Autodesk Fusion 360 part; units mm, degrees
(part 2 of 3)
  line L576 (512.1919, -690.0793) -> (454.1919, -690.0793)
  line L577 (454.1919, -748.0793) -> (512.1919, -690.0793) construction
  line L578 (527.085, -748.0793) -> (585.085, -748.0793)
  line L579 (512.1919, -748.0793) -> (454.1919, -690.0793) construction
  line L580 (513.1919, -749.0793) -> (526.085, -749.0793) construction
  line L581 (454.1919, -748.0793) -> (512.1919, -748.0793)
  line L582 (585.085, -748.0793) -> (585.085, -690.0793)
  line L583 (381.2987, -690.0793) -> (381.2987, -748.0793)
  line L584 (381.2987, -748.0793) -> (439.2987, -748.0793)
  line L585 (454.1919, -690.0793) -> (454.1919, -748.0793)
  line L586 (527.085, -748.0793) -> (585.085, -690.0793) construction
  line L587 (585.085, -690.0793) -> (527.085, -690.0793)
  line L588 (439.2987, -690.0793) -> (381.2987, -690.0793)
  line L589 (381.2987, -748.0793) -> (439.2987, -690.0793) construction
  line L590 (440.2987, -749.0793) -> (453.1919, -749.0793) construction
  line L591 (585.085, -748.0793) -> (527.085, -690.0793) construction
  line L592 (527.085, -690.0793) -> (527.085, -748.0793)
  line L593 (512.1919, -748.0793) -> (512.1919, -690.0793)
  line L594 (439.2987, -748.0793) -> (381.2987, -690.0793) construction
  line L595 (439.2987, -748.0793) -> (439.2987, -690.0793)
  line L596 (225.4513, -1098.8293) -> (283.4513, -1040.8293) construction
  line L597 (152.5581, -1098.8293) -> (152.5581, -1040.8293)
  line L598 (79.665, -1098.8293) -> (79.665, -1040.8293)
  line L599 (79.665, -1040.8293) -> (137.665, -1040.8293)
  line L600 (137.665, -1098.8293) -> (79.665, -1040.8293) construction
  line L601 (152.5581, -1040.8293) -> (210.5581, -1040.8293)
  line L602 (151.5581, -1099.8293) -> (138.665, -1099.8293) construction
  line L603 (137.665, -1040.8293) -> (137.665, -1098.8293)
  line L604 (79.665, -1098.8293) -> (137.665, -1040.8293) construction
  line L605 (152.5581, -1098.8293) -> (210.5581, -1040.8293) construction
  line L606 (210.5581, -1098.8293) -> (152.5581, -1098.8293)
  line L607 (210.5581, -1098.8293) -> (152.5581, -1040.8293) construction
  line L608 (137.665, -1098.8293) -> (79.665, -1098.8293)
  line L609 (210.5581, -1040.8293) -> (210.5581, -1098.8293)
  line L610 (225.4513, -1098.8293) -> (225.4513, -1040.8293)
  line L611 (283.4513, -1098.8293) -> (225.4513, -1098.8293)
  line L612 (225.4513, -1040.8293) -> (283.4513, -1040.8293)
  line L613 (283.4513, -1040.8293) -> (283.4513, -1098.8293)
  line L614 (283.4513, -1098.8293) -> (225.4513, -1040.8293) construction
  line L615 (224.4513, -1099.8293) -> (211.5581, -1099.8293) construction
  line L616 (332, -925) -> (332, -1216) construction
  line L617 (526.335, -1098.8293) -> (584.335, -1098.8293)
  line L618 (526.335, -1040.8293) -> (526.335, -1098.8293)
  line L619 (526.335, -1098.8293) -> (584.335, -1040.8293) construction
  line L620 (380.5487, -1040.8293) -> (380.5487, -1098.8293)
  line L621 (380.5487, -1098.8293) -> (438.5487, -1098.8293)
  line L622 (439.5487, -1099.8293) -> (452.4419, -1099.8293) construction
  line L623 (453.4419, -1040.8293) -> (453.4419, -1098.8293)
  line L624 (438.5487, -1098.8293) -> (380.5487, -1040.8293) construction
  line L625 (438.5487, -1098.8293) -> (438.5487, -1040.8293)
  line L626 (380.5487, -1098.8293) -> (438.5487, -1040.8293) construction
  line L627 (438.5487, -1040.8293) -> (380.5487, -1040.8293)
  line L628 (511.4419, -1098.8293) -> (511.4419, -1040.8293)
  line L629 (584.335, -1098.8293) -> (526.335, -1040.8293) construction
  line L630 (453.4419, -1098.8293) -> (511.4419, -1098.8293)
  line L631 (584.335, -1098.8293) -> (584.335, -1040.8293)
  line L632 (511.4419, -1098.8293) -> (453.4419, -1040.8293) construction
  line L633 (511.4419, -1040.8293) -> (453.4419, -1040.8293)
  line L634 (512.4419, -1099.8293) -> (525.335, -1099.8293) construction
  line L635 (584.335, -1040.8293) -> (526.335, -1040.8293)
  line L636 (453.4419, -1098.8293) -> (511.4419, -1040.8293) construction
  point P0 (-381.2407, -502.1425)
  point P1 (-1045.2407, -502.1425)
  point P2 (332, 4.5)
  point P3 (332, 4.5)
  point P4 (332, -345.5)
  point P5 (332, -345.5)
  point P6 (0, -350)
  point P7 (1200, -500)
  point P8 (1294, -456)
  point P9 (1200, -500)
  point P10 (1200, -412)
  point P11 (1388, -412)
  point P12 (1294, -456)
  point P13 (1755.9968, -408.7804)
  point P14 (1661.9968, -630.2804)
  point P15 (1661.9968, -630.2804)
  point P16 (1567.9968, -496.7804)
  point P17 (1661.9968, -452.7804)
  point P18 (1567.9968, -408.7804)
  point P19 (1661.9968, -452.7804)
  point P20 (1567.9968, -496.7804)
  point P21 (1661.9968, -452.7804)
  point P22 (1781.5009, -1445.9592)
  point P23 (2131.5009, -1445.9592)
  point P24 (2131.5009, -1095.9592)
  point P25 (1781.5009, -1095.9592)
  point P26 (861.9968, -1564.433)
  point P27 (861.9968, -1564.433)
  point P28 (166, -1297.5)
  point P29 (498, -1297.5)
  point P30 (166, -1297.5)
  point P31 (498, -1297.5)
  point P32 (501.8298, -1590.7079)
  point P33 (187.1704, -1945.0478)
  point P34 (501.8298, -1576.2079)
  point P35 (861.9968, -1548.433)
  point P36 (861.9968, -1562.933)
  point P37 (1211.9968, -1564.433)
  point P38 (1211.9968, -1548.433)
  point P39 (1211.9968, -1562.933)
  point P40 (1211.9968, -1564.433)
  point P41 (141.8298, -1576.2079)
  point P42 (141.8298, -1590.7079)
  point P43 (540.3102, -621.1975)
  point P44 (253.7013, -719.0793)
  point P45 (107.915, -719.0793)
  point P46 (123.6898, -621.1975)
  point P47 (107.915, -719.0793)
  point P48 (253.7013, -719.0793)
  point P49 (123.6898, -621.1975)
  point P50 (540.3102, -621.1975)
  point P51 (123.6898, -621.1975)
  point P52 (540.3102, -621.1975)
  point P53 (123.6898, -971.1975)
  point P54 (540.3102, -971.1975)
  point P55 (123.6898, -971.1975)
  point P56 (540.3102, -971.1975)
  point P57 (540.3102, -971.1975)
  point P58 (123.6898, -971.1975)
  point P59 (166, -1297.5)
  point P60 (312.5, -1297.5)
  point P61 (312.5, -1297.5)
  point P62 (107.915, -719.0793)
  point P63 (180.8081, -719.0793)
  point P64 (253.7013, -719.0793)
  point P65 (556.085, -719.0793)
  point P66 (410.2987, -719.0793)
  point P67 (556.085, -719.0793)
  point P68 (410.2987, -719.0793)
  point P69 (410.2987, -719.0793)
  point P70 (483.1919, -719.0793)
  point P71 (556.085, -719.0793)
  point P72 (79.665, -1040.8293)
  point P73 (181.5581, -1069.8293)
  point P74 (108.665, -1069.8293)
  point P75 (254.4513, -1069.8293)
  point P76 (254.4513, -1069.8293)
  point P77 (108.665, -1069.8293)
  point P78 (108.665, -1069.8293)
  point P79 (254.4513, -1069.8293)
  point P80 (482.4419, -1069.8293)
  point P81 (555.335, -1069.8293)
  point P82 (555.335, -1069.8293)
  point P83 (409.5487, -1069.8293)
  point P84 (584.335, -1040.8293)
  point P85 (555.335, -1069.8293)
  point P86 (409.5487, -1069.8293)
  point P87 (409.5487, -1069.8293)
  dimension "d11" = 7
  dimension "d12" = 16.1835
  dimension "d13" = 16.1835
  dimension "d14" = 16.1835
  dimension "d15" = 16.1835
  dimension "d16" = 11.9217
  dimension "d17" = 11.9217
  dimension "d19" = 11.9217
  dimension "d22" = 5.3
  dimension "d23" = 5.3
  dimension "d24" = 5.3
  dimension "d25" = 5.3
  dimension "d26" = 5.3
  dimension "d27" = 22
  dimension "d28" = 22
  dimension "d29" = 22
  dimension "d33" = 5.3
  dimension "d34" = 5.3
  dimension "d35" = 5.3
  dimension "d36" = 5.3
  dimension "d37" = 5.3
  dimension "d38" = 5.3
  dimension "d39" = 5.3
  dimension "d43" = 291
  dimension "d63" = 74.7336
  dimension "d64" = 86
  dimension "d65" = 43
  dimension "d83" = 12.8931
  dimension "d84" = 12.8931
  dimension "d85" = 60
  dimension "d89" = 7
  dimension "d90" = 16.1835
  dimension "d91" = 16.1835
  dimension "d92" = 16.1835
  dimension "d93" = 16.1835
  dimension "d94" = 11.9217
  dimension "d95" = 11.9217
  dimension "d96" = 11.9217
  dimension "d97" = 5.3
  dimension "d98" = 5.3
  dimension "d99" = 5.3
  dimension "d100" = 5.3
  dimension "d101" = 5.3
  dimension "d102" = 22
  dimension "d103" = 22
  dimension "d104" = 22
  dimension "d105" = 5.3
  dimension "d106" = 5.3
  dimension "d107" = 5.3
  dimension "d108" = 5.3
  dimension "d109" = 5.3
  dimension "d110" = 5.3
  dimension "d111" = 5.3
  dimension "d112" = 86
  dimension "d113" = 43
  dimension "d114" = 7
  dimension "d115" = 16.1835
  dimension "d116" = 16.1835
  dimension "d117" = 16.1835
  dimension "d118" = 16.1835
  dimension "d119" = 11.9217
  dimension "d120" = 11.9217
  dimension "d121" = 11.9217
  dimension "d122" = 5.3
  dimension "d123" = 5.3
  dimension "d124" = 5.3
  dimension "d125" = 5.3
  dimension "d126" = 5.3
  dimension "d127" = 22
  dimension "d128" = 22
  dimension "d129" = 22
  dimension "d130" = 5.3
  dimension "d131" = 5.3
  dimension "d132" = 5.3
  dimension "d133" = 5.3
  dimension "d134" = 5.3
  dimension "d135" = 5.3
  dimension "d136" = 5.3
  dimension "d137" = 86
  dimension "d138" = 43
  dimension "d194" = 73
  dimension "d195" = 664
  dimension "d196" = 73
  dimension "d203" = 7
  dimension "d204" = 5.3
  dimension "d205" = 5.3
  dimension "d206" = 5.3
  dimension "d207" = 5.3
  dimension "d208" = 5.3
  dimension "d209" = 5.3
  dimension "d210" = 5.3
  dimension "d211" = 5.3
  dimension "d212" = 5.3
  dimension "d213" = 5.3
  dimension "d214" = 5.3
  dimension "d215" = 5.3
  dimension "d216" = 291
  dimension "d217" = 33
  dimension "d218" = 332
  dimension "d219" = 60
  dimension "d220" = 664
  dimension "d350" = 291
  dimension "d352" = 231
  dimension "d357" = 28.284
  dimension "d358" = 28.284
  dimension "d359" = 28.284
  dimension "d360" = 28.284
  dimension "d361" = 664
  dimension "d362" = 291
  dimension "d363" = 231
  dimension "d364" = 28.284
  dimension "d365" = 28.284
  dimension "d366" = 28.284
  dimension "d367" = 28.284
  dimension "d368" = 30
  dimension "d369" = 30
  dimension "d370" = 30
  dimension "d371" = 30
  dimension "d372" = 30
  dimension "d373" = 30
  dimension "d374" = 30
  dimension "d375" = 30
  dimension "d376" = 6.5
  dimension "d377" = 6.5
  dimension "d378" = 18
  dimension "d379" = 18
  dimension "d380" = 18
  dimension "d381" = 18
  dimension "d382" = 6.5
  dimension "d383" = 6.5
  dimension "d384" = 20
  dimension "d385" = 20
  dimension "d387" = 20
  dimension "d389" = 20
  dimension "d390" = 20
  dimension "d391" = 20
  dimension "d392" = 5
  dimension "d393" = 5
  dimension "d394" = 5
  dimension "d395" = 5
  dimension "d537" = 664
  dimension "d553" = 67
  dimension "d554" = 67
  dimension "d555" = 67
  dimension "d556" = 67
  dimension "d1" = 188
  dimension "d2" = 88
  dimension "d3" = 18
  dimension "d4" = 18
  dimension "d5" = 18
  dimension "d6" = 18
  dimension "d7" = 15
  dimension "d8" = 15
  dimension "d9" = 15
  dimension "d10" = 15
  dimension "d597" = 8
  dimension "d598" = 8
  dimension "d599" = 8
  dimension "d600" = 8
  dimension "d601" = 8
  dimension "d602" = 8
  dimension "d603" = 8
  dimension "d604" = 8
  dimension "d605" = 73
  dimension "d606" = 80
  dimension "d607" = 188
  dimension "d608" = 88
  dimension "d609" = 18
  dimension "d610" = 18
  dimension "d611" = 18
  dimension "d612" = 18
  dimension "d613" = 15
  dimension "d614" = 15
  dimension "d615" = 15
  dimension "d616" = 15
  dimension "d617" = 25
  dimension "d618" = 25
  dimension "d807" = 300
  dimension "d858" = 30
  dimension "d859" = 30
  dimension "d860" = 30
  dimension "d861" = 30
  dimension "d862" = 6.5
  dimension "d863" = 6.5
  dimension "d865" = 6.5
  dimension "d876" = 30
  dimension "d877" = 30
  dimension "d878" = 30
  dimension "d879" = 30
  dimension "d880" = 20
  dimension "d881" = 20
  dimension "d882" = 20
  dimension "d883" = 20
  dimension "d884" = 6.5
  dimension "d892" = 30
  dimension "d893" = 30
  dimension "d894" = 30
  dimension "d895" = 30
  dimension "d896" = 6.5
  dimension "d897" = 6.5
  dimension "d898" = 6.5
  dimension "d899" = 30
  dimension "d900" = 30
  dimension "d901" = 30
  dimension "d902" = 30
  dimension "d903" = 20
  dimension "d904" = 20
  dimension "d905" = 20
  dimension "d906" = 20
  dimension "d907" = 6.5
  dimension "d934" = 300
  dimension "d943" = 25
  dimension "d944" = 25
  dimension "d945" = 20
  dimension "d946" = 20
  dimension "d947" = 20
  dimension "d948" = 20
  dimension "d949" = 20
  dimension "d950" = 20
  dimension "d951" = 20
  dimension "d953" = 5
  dimension "d954" = 5
  dimension "d955" = 5
  dimension "d956" = 5
  dimension "d957" = 300
  dimension "d959" = 20
  dimension "d961" = 20
  dimension "d962" = 20
  dimension "d963" = 20
  dimension "d964" = 20
  dimension "d965" = 20
  dimension "d966" = 5
  dimension "d967" = 5
  dimension "d968" = 5
  dimension "d969" = 5
  dimension "d981" = 37.5
  dimension "d983" = 37.5
  dimension "d1011" = 8
  dimension "d1012" = 8
  dimension "d1013" = 8
  dimension "d1014" = 8
  dimension "d1015" = 8
  dimension "d1016" = 8
  dimension "d1017" = 8
  dimension "d1018" = 29
  dimension "d1019" = 45.5
  dimension "d1020" = 22
  dimension "d1037" = 8
  dimension "d1038" = 8
  dimension "d1039" = 8
  dimension "d1040" = 8
  dimension "d1041" = 8
  dimension "d1042" = 8
  dimension "d1043" = 8
  dimension "d1044" = 29
  dimension "d1045" = 45.5
  dimension "d1046" = 22
  dimension "d1047" = 45.5
  dimension "d1048" = 26.5
  dimension "d1049" = 182
  dimension "d1050" = 29
  dimension "d1051" = 45.5
  dimension "d1052" = 22
  dimension "d1055" = 2.5
  dimension "d1056" = 1.9
  dimension "d1057" = 273
  dimension "d1058" = 73
  dimension "d1059" = 8
  dimension "d1060" = 8
  dimension "d1061" = 8
  dimension "d1062" = 8
  dimension "d1063" = 8
  dimension "d1064" = 8
  dimension "d1065" = 8
  dimension "d1066" = 29
  dimension "d1069" = 182
  dimension "d1072" = 2.5
  dimension "d1073" = 1.9
  dimension "d1074" = 54.5
  dimension "d1075" = 26.5
  dimension "d1076" = 54.5
  dimension "d1077" = 17.5
  dimension "d1094" = 25
  dimension "d1095" = 25
  dimension "d1096" = 8
  dimension "d1097" = 8
  dimension "d1098" = 8
  dimension "d1099" = 8
  dimension "d1100" = 8
  dimension "d1101" = 8
  dimension "d1102" = 8
  dimension "d1103" = 29
  dimension "d1104" = 182
  dimension "d1105" = 2.5
  dimension "d1106" = 1.9
  dimension "d1107" = 54.5
  dimension "d1108" = 26.5
  dimension "d1109" = 54.5
  dimension "d1110" = 26.5
  dimension "d1111" = 8
  dimension "d1112" = 8
  dimension "d1113" = 8
  dimension "d1114" = 8
  dimension "d1115" = 8
  dimension "d1116" = 8
  dimension "d1117" = 8
  dimension "d1118" = 29
  dimension "d1119" = 45.5
  dimension "d1120" = 22
  dimension "d1121" = 182
  dimension "d1122" = 45.5
  dimension "d1123" = 22
  dimension "d1124" = 2.5
  dimension "d1125" = 1.9
  dimension "d1126" = 273
  dimension "d1127" = 73
  dimension "d1144" = 29
  dimension "d1145" = 29
  dimension "d1146" = 29
  dimension "d1147" = 29
  dimension "d1148" = 7
  dimension "d1171" = 291
  dimension "d1174" = 74.7336
  dimension "d1187" = 20
  dimension "d1188" = 20
  dimension "d1189" = 20
  dimension "d1190" = 20
  dimension "d1191" = 20
  dimension "d1192" = 20
  dimension "d1193" = 5
  dimension "d1194" = 5
  dimension "d1195" = 5
  dimension "d1196" = 5
  dimension "d1197" = 664
  dimension "d1210" = 29
  dimension "d1211" = 29
  dimension "d1212" = 29
  dimension "d1213" = 29
  dimension "d1237" = 291
  dimension "d1253" = 20
  dimension "d1254" = 20
  dimension "d1255" = 20
  dimension "d1256" = 20
  dimension "d1257" = 20
  dimension "d1258" = 20
  dimension "d1259" = 5
  dimension "d1260" = 5
  dimension "d1261" = 5
  dimension "d1262" = 5
  dimension "d1263" = 664
  dimension "d1322" = 29
  dimension "d1323" = 29
  dimension "d1324" = 12.5
  dimension "d1325" = 12.5
  dimension "d1326" = 58
  dimension "d1327" = 58
  dimension "d1328" = 58
  dimension "d1329" = 58
  dimension "d1330" = 58
  dimension "d1331" = 58
  dimension "d1332" = 12.8931
  dimension "d1333" = 12.8931
  dimension "d1334" = 60
  dimension "d1335" = 58
  dimension "d1336" = 58
  dimension "d1337" = 58
  dimension "d1338" = 58
  dimension "d1339" = 58
  dimension "d1340" = 58
  constraint horizontal L0
  constraint horizontal L1
  constraint tangent L0 A0
  constraint tangent L1 A0
  constraint tangent L0 A1
  constraint tangent L1 A1
  constraint coincident L0.end A1.end
  constraint vertical L5
  constraint parallel L5 L6
  constraint parallel L6 L7
  constraint vertical L14
  constraint parallel L9 L14
  constraint parallel L9 L13
  constraint tangent A1 L15
  constraint horizontal L16
  constraint vertical L17
  constraint horizontal L19
  constraint vertical L20
  constraint coincident L17.end L18.start
  constraint coincident L20.end L21.end
  constraint coincident L4.end L5.start
  constraint coincident L7.end L8.end
  constraint coincident L22.start A7.centre
  constraint horizontal L23
  constraint parallel L23 L24
  constraint parallel L24 L25
  constraint horizontal L27
  constraint parallel L27 L28
  constraint parallel L28 L29
  constraint coincident L23.end L24.start
  constraint coincident L24.end L25.start
  constraint coincident L25.end A10.centre
  constraint coincident L26.start L27.start
  constraint coincident L27.end L28.start
  constraint coincident L28.end L29.start
  constraint coincident L29.end A14.centre
  constraint horizontal L30
  constraint vertical L31
  constraint horizontal L32
  constraint vertical L33
  constraint horizontal L34
  constraint vertical L35
  constraint vertical L36
  constraint perpendicular L35 L37
  constraint coincident A0.centre L37.end
  constraint horizontal L51
  constraint horizontal L53
  constraint tangent L51 A29
  constraint tangent L53 A29
  constraint tangent A22 L51
  constraint tangent A22 L53
  constraint coincident L42.start A20.end
  constraint vertical L67
  constraint parallel L40 L67
  constraint parallel L40 L44
  constraint vertical L65
  constraint parallel L65 L68
  constraint parallel L66 L68
  constraint tangent L47 A22
  constraint horizontal L56
  constraint vertical L54
  constraint horizontal L60
  constraint vertical L61
  constraint coincident L54.end L58.start
  constraint coincident A27.centre L61.end
  constraint coincident A19.centre L64.end
  constraint coincident L41.end L43.end
  constraint coincident L57.start A26.centre
  constraint horizontal L57
  constraint parallel L52 L57
  constraint parallel L45 L52
  constraint horizontal L46
  constraint parallel L46 L50
  constraint parallel L50 L59
  constraint coincident L52.start L57.end
  constraint coincident A16.centre L45.start
  constraint coincident L45.end A21.centre
  constraint coincident L41.start A17.centre
  constraint coincident A15.centre L46.end
  constraint coincident L50.end A24.centre
  constraint coincident A23.centre L59.end
  constraint coincident L55.end A29.centre
  constraint horizontal L81
  constraint horizontal L79
  constraint tangent A32 L81
  constraint tangent A32 L79
  constraint tangent L81 A37
  constraint tangent L79 A37
  constraint coincident L81.end A37.end
  constraint vertical L71
  constraint parallel L71 L80
  constraint parallel L80 L92
  constraint vertical L88
  constraint parallel L88 L100
  constraint parallel L91 L100
  constraint tangent A37 L84
  constraint horizontal L78
  constraint vertical L93
  constraint horizontal L74
  constraint vertical L75
  constraint coincident A33.centre L93.end
  constraint coincident L72.end L75.end
  constraint coincident L71.start L82.end
  constraint coincident A30.centre L86.end
  constraint coincident L76.start A43.centre
  constraint horizontal L76
  constraint parallel L73 L76
  constraint parallel L73 L85
  constraint horizontal L90
  constraint parallel L90 L95
  constraint parallel L95 L97
  constraint coincident L73.start L76.end
  constraint coincident L73.end L85.start
  constraint coincident A31.centre L85.end
  constraint coincident A36.centre L87.start
  constraint coincident A40.centre L90.end
  constraint coincident L95.end L97.start
  constraint coincident A34.centre L97.end
  constraint coincident A32.centre L96.end
  constraint horizontal L102
  constraint vertical L103
  constraint horizontal L104
  constraint vertical L105
  constraint horizontal L108
  constraint vertical L107
  constraint horizontal L109
  constraint vertical L106
  constraint horizontal L128
  constraint horizontal L127
  constraint tangent A50 L128
  constraint tangent A50 L127
  constraint tangent L128 A59
  constraint tangent L127 A59
  constraint horizontal L136
  constraint vertical L152
  constraint horizontal L139
  constraint vertical L140
  constraint vertical L121
  constraint vertical L129
  constraint horizontal L135
  constraint vertical L130
  constraint horizontal L131
  constraint vertical L138
  constraint horizontal L149
  constraint vertical L142
  constraint horizontal L150
  constraint vertical L147
  constraint horizontal L137
  constraint vertical L134
  constraint horizontal L145
  constraint vertical L143
  constraint horizontal L146
  constraint vertical L151
  constraint perpendicular L143 L144
  constraint horizontal L119
  constraint vertical L126
  constraint horizontal L114
  constraint vertical L148
  constraint perpendicular L111 L126
  constraint horizontal L110
  constraint vertical L154
  constraint horizontal L153
  constraint vertical L155
  constraint horizontal L115
  constraint vertical L117
  constraint horizontal L113
  constraint vertical L124
  constraint horizontal L132
  constraint vertical L112
  constraint horizontal L141
  constraint vertical L123
  constraint horizontal L120
  constraint vertical L125
  constraint horizontal L116
  constraint vertical L122
  constraint horizontal L164
  constraint vertical L156
  constraint horizontal L158
  constraint vertical L157
  constraint horizontal L159
  constraint perpendicular L159 L161
  constraint parallel L159 L163
  constraint parallel L160 L161
  constraint coincident P3 L162
  constraint coincident P3 L165
  constraint coincident P3 P2
  constraint vertical L166
  constraint horizontal L176
  constraint vertical L174
  constraint horizontal L178
  constraint vertical L183
  constraint horizontal L182
  constraint perpendicular L180 L182
  constraint parallel L177 L182
  constraint parallel L173 L180
  constraint coincident P5 L179
  constraint coincident P5 L175
  constraint coincident P5 P4
  constraint vertical L185
  constraint coincident L165.start L159
  constraint coincident L165.start L161
  constraint tangent L159 A60
  constraint tangent L161 A60
  constraint coincident L162.start L159
  constraint coincident L162.start L160
  constraint tangent L159 A61
  constraint tangent L160 A61
  constraint coincident L165.end L160
  constraint coincident L165.end L163
  constraint tangent L160 A62
  constraint tangent L163 A62
  constraint coincident L162.end L161
  constraint coincident L162.end L163
  constraint tangent L161 A63
  constraint tangent L163 A63
  constraint coincident L175.start L182
  constraint coincident L175.start L180
  constraint tangent L182 A64
  constraint tangent L180 A64
  constraint coincident L179.start L182
  constraint coincident L179.start L173
  constraint tangent L182 A65
  constraint tangent L173 A65
  constraint coincident L175.end L173
  constraint coincident L175.end L177
  constraint tangent L173 A66
  constraint tangent L177 A66
  constraint coincident L179.end L180
  constraint coincident L179.end L177
  constraint tangent L180 A67
  constraint tangent L177 A67
  constraint coincident L172.end A68.centre
  constraint coincident L171.end A69.centre
  constraint coincident L167.end A70.centre
  constraint coincident L168.end A71.centre
  constraint coincident L169.end A72.centre
  constraint coincident L170.end A73.centre
  constraint coincident L184.end A74.centre
  constraint coincident L181.end A75.centre
  constraint horizontal L186
  constraint vertical L187
  constraint horizontal L188
  constraint vertical L189
  constraint horizontal L190
  constraint vertical L191
  constraint horizontal L192
  constraint vertical L193
  constraint horizontal L194
  constraint vertical L195
  constraint horizontal L196
  constraint vertical L197
  constraint horizontal L198
  constraint vertical L199
  constraint horizontal L200
  constraint vertical L201
  constraint coincident L199.end L200.start
  constraint coincident L187.end L188.start
  constraint coincident L195.end L196.start
  constraint coincident L191.end L192.start
  constraint horizontal L202
  constraint vertical L203
  constraint horizontal L204
  constraint vertical L205
  constraint horizontal L206
  constraint vertical L207
  constraint horizontal L208
  constraint vertical L209
  constraint horizontal L210
  constraint vertical L211
  constraint horizontal L212
  constraint vertical L213
  constraint horizontal L214
  constraint vertical L215
  constraint horizontal L216
  constraint vertical L217
  constraint horizontal L218
  constraint vertical L219
  constraint horizontal L220
  constraint vertical L221
  constraint horizontal L224
  constraint vertical L225
  constraint horizontal L222
  constraint vertical L223
  constraint horizontal L231
  constraint vertical L233
  constraint horizontal L232
  constraint vertical L230
  constraint horizontal L227
  constraint vertical L228
  constraint horizontal L229
  constraint vertical L226
  constraint horizontal L239
  constraint vertical L247
  constraint horizontal L245
  constraint vertical L250
  constraint coincident P9 P7
  constraint horizontal L234
  constraint vertical L252
  constraint horizontal L253
  constraint vertical L249
  constraint horizontal L235
  constraint vertical L236
  constraint horizontal L241
  constraint vertical L248
  constraint coincident P10 L245
  constraint coincident P10 L250
  constraint tangent A82 L245
  constraint tangent A82 L250
  constraint coincident P9 L250
  constraint coincident P9 L239
  constraint tangent A89 L250
  constraint tangent L239 A89
  constraint coincident P11 L245
  constraint coincident P11 L247
  constraint tangent A85 L245
  constraint tangent A85 L247
  constraint tangent L247 A88
  constraint tangent L239 A88
  constraint coincident P11 L240.start
  constraint coincident P10 L242.start
  constraint midpoint P12 L240
  constraint horizontal L244
  constraint perpendicular L243 L244
  constraint parallel L238 L244
  constraint parallel L243 L251
  constraint coincident P12 L246
  constraint coincident P12 L237
  constraint coincident P12 P8
  constraint coincident L246.start L244
  constraint coincident L246.start L251
  constraint tangent L244 A90
  constraint tangent A90 L251
  constraint coincident L237.end L251
  constraint coincident L237.end L238
  constraint tangent A80 L251
  constraint tangent A80 L238
  constraint coincident L237.start L244
  constraint coincident L237.start L243
  constraint tangent A83 L244
  constraint tangent A83 L243
  constraint coincident L246.end L243
  constraint coincident L246.end L238
  constraint tangent A84 L243
  constraint tangent A84 L238
  constraint vertical L285
  constraint vertical L284
  constraint horizontal L287
  constraint vertical L272
  constraint coincident P15 P14
  constraint perpendicular L284 L286
  constraint perpendicular L273 L285
  constraint horizontal L283
  constraint vertical L271
  constraint horizontal L280
  constraint vertical L261
  constraint perpendicular L264 L280
  constraint coincident L282.end L285
  constraint horizontal L274
  constraint vertical L270
  constraint horizontal L281
  constraint vertical L260
  constraint coincident P20 P16
  constraint horizontal L268
  constraint vertical L269
  constraint horizontal L266
  constraint vertical L263
  constraint horizontal L254
  constraint vertical L259
  constraint horizontal L258
  constraint vertical L257
  constraint coincident P18 L281
  constraint coincident P18 L260
  constraint tangent A93 L281
  constraint tangent A93 L260
  constraint coincident P20 L260
  constraint coincident P20 L274
  constraint tangent L260 A107
  constraint tangent L274 A107
  constraint coincident P13 L281
  constraint coincident P13 L270
  constraint tangent A99 L281
  constraint tangent A99 L270
  constraint tangent A101 L270
  constraint tangent A101 L274
  constraint horizontal L276
  constraint perpendicular L256 L276
  constraint parallel L275 L276
  constraint parallel L256 L267
  constraint coincident P21 P19
  constraint tangent A97 L276
  constraint tangent A97 L267
  constraint tangent A100 L267
  constraint tangent A100 L275
  constraint tangent A103 L276
  constraint tangent L256 A103
  constraint tangent L256 A108
  constraint tangent L275 A108
  constraint midpoint P21 L279
  constraint horizontal L277
  constraint midpoint A94.centre L278
  constraint midpoint A96.centre L265
  constraint vertical L293
  constraint vertical L291
  constraint horizontal L289
  constraint perpendicular L290 L291
  constraint perpendicular L288 L293
  constraint horizontal L292
  constraint vertical L296
  constraint vertical L303
  constraint horizontal L294
  constraint perpendicular L294 L295
  constraint parallel L294 L305
  constraint parallel L295 L304
  constraint tangent L294 A115
  constraint tangent A115 L295
  constraint tangent L294 A127
  constraint tangent L304 A127
  constraint tangent A114 L295
  constraint tangent A114 L305
  constraint tangent L304 A126
  constraint tangent L305 A126
  constraint vertical L302
  constraint vertical L299
  constraint horizontal L297
  constraint perpendicular L297 L301
  constraint parallel L297 L298
  constraint parallel L300 L301
  constraint tangent L297 A125
  constraint tangent A125 L301
  constraint tangent A118 L297
  constraint tangent A118 L300
  constraint tangent A124 L301
  constraint tangent L298 A124
  constraint tangent A119 L300
  constraint tangent A119 L298
  constraint horizontal L306
  constraint horizontal L307
  constraint horizontal L308
  constraint horizontal L309
  constraint vertical L313
  constraint vertical L311
  constraint horizontal L319
  constraint perpendicular L312 L319
  constraint parallel L317 L319
  constraint parallel L312 L318
  constraint tangent L319 A137
  constraint tangent L312 A137
  constraint tangent A130 L319
  constraint tangent A130 L318
  constraint tangent L312 A136
  constraint tangent L317 A136
  constraint tangent L318 A134
  constraint tangent L317 A134
  constraint vertical L320
  constraint vertical L314
  constraint horizontal L325
  constraint perpendicular L322 L325
  constraint parallel L315 L325
  constraint parallel L322 L324
  constraint tangent A141 L325
  constraint tangent L322 A141
  constraint tangent L325 A145
  constraint tangent L324 A145
  constraint tangent A138 L322
  constraint tangent L315 A138
  constraint tangent L324 A144
  constraint tangent L315 A144
  constraint horizontal L321
  constraint horizontal L310
  constraint horizontal L323
  constraint horizontal L316
  constraint vertical L326
  constraint vertical L330
  constraint horizontal L331
  constraint vertical L329
  constraint horizontal L327
  constraint horizontal L328
  constraint horizontal L332
  constraint vertical L333
  constraint horizontal L334
  constraint vertical L335
  constraint horizontal L336
  constraint vertical L337
  constraint horizontal L338
  constraint vertical L339
  constraint horizontal L340
  constraint vertical L341
  constraint horizontal L342
  constraint vertical L343
  constraint horizontal L344
  constraint vertical L345
  constraint horizontal L346
  constraint vertical L347
  constraint coincident L345.end L346.start
  constraint coincident L333.end L334.start
  constraint coincident L337.end L338.start
  constraint coincident L341.end L342.start
  constraint vertical L349
  constraint vertical L366
  constraint horizontal L362
  constraint perpendicular L356 L366
  constraint perpendicular L349 L368
  constraint horizontal L365
  constraint horizontal L355
  constraint vertical L348
  constraint horizontal L354
  constraint vertical L353
  constraint horizontal L367
  constraint vertical L369
  constraint horizontal L352
  constraint vertical L359
  constraint horizontal L364
  constraint vertical L361
  constraint horizontal L351
  constraint vertical L360
  constraint horizontal L358
  constraint vertical L363
  constraint horizontal L357
  constraint vertical L350
  constraint coincident A156.centre L357.start
  constraint coincident L348.end L354.start
  constraint coincident L352.start A158.centre
  constraint coincident L351.start L361.end
  constraint horizontal L370
  constraint vertical L371
  constraint horizontal L372
  constraint vertical L373
  constraint horizontal L374
  constraint vertical L375
  constraint horizontal L376
  constraint vertical L377
  constraint coincident P59 P30
  constraint coincident P31 P29
  constraint coincident P32 A165.centre
  constraint horizontal L379
  constraint vertical L378
  constraint horizontal L385
  constraint vertical L383
  constraint horizontal L381
  constraint vertical L380
  constraint horizontal L384
  constraint vertical L382
  constraint coincident P33 A173.centre
  constraint horizontal L389
  constraint vertical L391
  constraint horizontal L387
  constraint vertical L396
  constraint horizontal L395
  constraint vertical L386
  constraint horizontal L397
  constraint vertical L388
  constraint horizontal L390
  constraint vertical L392
  constraint horizontal L394
  constraint vertical L393
  constraint horizontal L398
  constraint vertical L399
  constraint horizontal L400
  constraint vertical L401
  constraint horizontal L402
  constraint perpendicular L402 L403
  constraint parallel L402 L404
  constraint parallel L403 L405
  constraint midpoint L379 P34
  constraint tangent L405 A174
  constraint tangent L402 A174
  constraint tangent L405 A175
  constraint tangent L404 A175
  constraint equal A174 A175
  constraint tangent L403 A176
  constraint tangent L404 A176
  constraint equal A174 A176
  constraint tangent L402 A177
  constraint tangent L403 A177
  constraint horizontal L406
  constraint vertical L407
  constraint horizontal L408
  constraint vertical L409
  constraint coincident P36 A182.centre
  constraint horizontal L416
  constraint vertical L417
  constraint horizontal L414
  constraint vertical L411
  constraint horizontal L412
  constraint perpendicular L412 L415
  constraint parallel L412 L413
  constraint parallel L410 L415
  constraint midpoint P35 L416
  constraint tangent A178 L410
  constraint tangent A178 L412
  constraint tangent L410 A179
  constraint tangent A179 L413
  constraint equal A178 A179
  constraint tangent A180 L415
  constraint tangent A180 L413
  constraint equal A178 A180
  constraint tangent L412 A183
  constraint tangent A183 L415
  constraint horizontal L418
  constraint vertical L419
  constraint horizontal L420
  constraint vertical L421
  constraint horizontal L422
  constraint vertical L423
  constraint horizontal L424
  constraint vertical L425
  constraint vertical L443
  constraint vertical L432
  constraint horizontal L447
  constraint vertical L441
  constraint horizontal L445
  constraint horizontal L438
  constraint coincident P39 A193.centre
  constraint horizontal L446
  constraint vertical L431
  constraint horizontal L444
  constraint vertical L427
  constraint horizontal L428
  constraint perpendicular L428 L436
  constraint parallel L428 L437
  constraint parallel L435 L436
  constraint midpoint P38 L446
  constraint tangent A192 L435
  constraint tangent A192 L428
  constraint tangent A191 L435
  constraint tangent A191 L437
  constraint equal A191 A192
  constraint tangent A195 L436
  constraint tangent A195 L437
  constraint equal A192 A195
  constraint tangent L428 A199
  constraint tangent A199 L436
  constraint horizontal L433
  constraint vertical L434
  constraint horizontal L426
  constraint vertical L430
  constraint horizontal L439
  constraint vertical L442
  constraint horizontal L440
  constraint vertical L429
  constraint coincident P42 A211.centre
  constraint horizontal L451
  constraint vertical L454
  constraint horizontal L460
  constraint vertical L465
  constraint horizontal L461
  constraint vertical L467
  constraint horizontal L464
  constraint vertical L463
  constraint horizontal L457
  constraint vertical L455
  constraint horizontal L448
  constraint vertical L456
  constraint horizontal L450
  constraint perpendicular L450 L452
  constraint parallel L449 L450
  constraint parallel L452 L458
  constraint midpoint P41 L451
  constraint tangent L458 A212
  constraint tangent L450 A212
  constraint tangent A206 L458
  constraint tangent L449 A206
  constraint equal A206 A212
  constraint tangent L452 A207
  constraint tangent L449 A207
  constraint equal A207 A212
  constraint tangent L450 A209
  constraint tangent L452 A209
  constraint horizontal L466
  constraint vertical L453
  constraint horizontal L459
  constraint vertical L462
  constraint coincident P62 P47
  constraint coincident P64 P48
  constraint coincident P51 P49
  constraint coincident P52 P50
  constraint horizontal L468
  constraint perpendicular L468 L469
  constraint parallel L468 L470
  constraint parallel L469 L471
  constraint coincident L472 P51
  constraint coincident L473 P51
  constraint horizontal L474
  constraint perpendicular L474 L475
  constraint parallel L474 L476
  constraint parallel L475 L477
  constraint coincident L478 P52
  constraint coincident L479 P52
  constraint horizontal L512
  constraint horizontal L509
  constraint tangent A220 L512
  constraint tangent A220 L509
  constraint tangent A221 L512
  constraint tangent A221 L509
  constraint horizontal L511
  constraint vertical L495
  constraint horizontal L510
  constraint vertical L497
  constraint horizontal L500
  constraint vertical L490
  constraint horizontal L485
  constraint vertical L496
  constraint horizontal L481
  constraint vertical L494
  constraint horizontal L480
  constraint vertical L482
  constraint horizontal L513
  constraint vertical L514
  constraint horizontal L501
  constraint vertical L504
  constraint horizontal L502
  constraint vertical L503
  constraint horizontal L487
  constraint vertical L488
  constraint horizontal L506
  constraint vertical L498
  constraint coincident L488.end A223.centre
  constraint coincident L481.start A218.centre
  constraint coincident A219.centre L502.start
  constraint coincident A217.centre L482.end
  constraint coincident P58 P55
  constraint coincident P57 P56
  constraint horizontal L505
  constraint perpendicular L486 L505
  constraint parallel L499 L505
  constraint parallel L486 L489
  constraint coincident P58 L508
  constraint coincident P58 L507
  constraint horizontal L493
  constraint perpendicular L484 L493
  constraint parallel L493 L515
  constraint parallel L484 L491
  constraint coincident P57 L492
  constraint coincident P57 L483
  constraint horizontal L526
  constraint vertical L524
  constraint horizontal L527
  constraint vertical L528
  constraint horizontal L525
  constraint horizontal L517
  constraint vertical L516
  constraint horizontal L518
  constraint vertical L520
  constraint horizontal L522
  constraint vertical L521
  constraint horizontal L523
  constraint vertical L519
  constraint horizontal L532
  constraint vertical L529
  constraint horizontal L530
  constraint vertical L531
  constraint horizontal L533
  constraint vertical L535
  constraint horizontal L534
  constraint vertical L536
  constraint coincident A227.centre L534.start
  constraint coincident L516.end L518.start
  constraint coincident L529.end L530.start
  constraint coincident A224.centre L521.end
  constraint horizontal L537
  constraint perpendicular L537 L538
  constraint parallel L537 L539
  constraint parallel L538 L540
  constraint coincident L541 P59
  constraint coincident L542 P59
  constraint horizontal L543
  constraint perpendicular L543 L544
  constraint parallel L543 L545
  constraint parallel L544 L546
  constraint coincident L547 P61
  constraint coincident L548 P61
  constraint coincident P61 P60
  constraint midpoint L104 L549.start
  constraint midpoint L102 L549.end
  constraint symmetric L537.start L549 L550.start
  constraint symmetric L537.end L549 L550.end
  constraint symmetric L538.end L549 L551.end
  constraint symmetric L539.end L549 L552.start
  constraint symmetric L543.start L549 L556.start
  constraint symmetric L543.end L549 L554.start
  constraint symmetric L544.end L549 L554.end
  constraint symmetric L545.end L549 L555.end
  constraint horizontal L558
  constraint perpendicular L558 L559
  constraint parallel L558 L560
  constraint parallel L559 L561
  constraint coincident L562 P62
  constraint coincident L563 P62
  constraint horizontal L564
  constraint perpendicular L564 L565
  constraint parallel L564 L566
  constraint parallel L565 L567
  constraint coincident L568 P63
  constraint coincident L569 P63
  constraint horizontal L570
  constraint perpendicular L570 L571
  constraint parallel L570 L572
  constraint parallel L571 L573
  constraint coincident L574 P64
  constraint coincident L575 P64
  constraint symmetric L35 L38.end L580.end
  constraint symmetric L35 L38.start L580.start
  constraint symmetric L35 L39.start L590.start
  constraint symmetric L35 L39.end L590.end
  constraint symmetric L35 P64 P69
  constraint symmetric L35 P62 P71
  constraint symmetric L35 L558.start L578.start
  constraint symmetric L35 L558.end L578.end
  constraint symmetric L35 L559.end L582.end
  constraint symmetric L35 L560.end L587.end
  constraint symmetric L35 L564.start L577.start
  constraint symmetric L35 L564.end L579.start
  constraint symmetric L35 L565.end L576.start
  constraint symmetric L35 L566.end L576.end
  constraint symmetric L35 P63 P70
  constraint symmetric L35 L570.start L583.end
  constraint symmetric L35 L570.end L584.end
  constraint symmetric L35 L571.end L588.start
  constraint symmetric L35 L572.end L583.start
  constraint coincident P78 P77
  constraint coincident P79 P76
  constraint horizontal L608
  constraint perpendicular L598 L608
  constraint parallel L599 L608
  constraint parallel L598 L603
  constraint coincident P78 L600
  constraint coincident P78 L604
  constraint horizontal L606
  constraint perpendicular L597 L606
  constraint parallel L601 L606
  constraint parallel L597 L609
  constraint coincident P73 L607
  constraint coincident P73 L605
  constraint horizontal L611
  constraint perpendicular L610 L611
  constraint parallel L611 L612
  constraint parallel L610 L613
  constraint coincident P79 L614
  constraint coincident P79 L596
  constraint coincident P72 L598.end
  constraint midpoint L510 L616.end
  constraint perpendicular L510 L616
  constraint symmetric P72 L616 P84
  constraint symmetric L602.start L616 L634.start
  constraint symmetric L602.end L616 L634.end
  constraint symmetric L615.start L616 L622.start
  constraint symmetric L615.end L616 L622.end
  constraint symmetric L597.start L616 L628.start
  constraint symmetric L596.end L616 L620.start
  constraint symmetric L596.start L616 L621.end
  constraint symmetric L606.start L616 L623.end
  constraint symmetric L611.start L616 L620.end
  constraint symmetric L601.end L616 L623.start
  constraint symmetric P73 L616 P80
  constraint symmetric P78 L616 P85
  constraint symmetric L597.end L616 L628.end
  constraint symmetric L600.start L616 L617.start
  constraint symmetric L599.end L616 L618.start
  constraint symmetric P79 L616 P87
  constraint symmetric L598.start L616 L617.end
  constraint symmetric L610.end L616 L625.end
  measures "d11" radius of A0
  measures "d12" distance of L4.end L5.end
  measures "d13" distance of L6.end L7.end
  measures "d14" distance of L5.end L4.end
  measures "d15" distance of L6.end L7.end
  measures "d16" distance of L0.end L15.end
  measures "d17" distance of L0.start L16.end
  measures "d19" distance of L1.end L19.end
  measures "d22" diameter of A3
  measures "d23" diameter of A4
  measures "d24" diameter of A5
  measures "d25" diameter of A6
  measures "d26" diameter of A7
  measures "d27" distance of L22.start L23.end
  measures "d28" distance of L23.end L24.end
  measures "d29" distance of L24.end L25.end
  measures "d33" diameter of A8
  measures "d34" diameter of A9
  measures "d35" diameter of A10
  measures "d36" diameter of A11
  measures "d37" diameter of A12
  measures "d38" diameter of A13
  measures "d39" diameter of A14
  measures "d43" distance of L30.start L32.end
  measures "d63" distance of L30.start L36.start
  measures "d64" distance of A0.centre A1.centre
  measures "d65" distance of L35.end A0.centre
  measures "d83" distance of L38.end L38.start
  measures "d84" distance of L39.start L39.end
  measures "d85" distance of L38.start L39.end
  measures "d89" radius of A29
  measures "d90" distance of L40.start A19.centre
  measures "d91" distance of L40.end L41.end
  measures "d92" distance of L40.start A19.centre
  measures "d93" distance of L40.end L41.end
  measures "d94" distance of L42.start L47.end
  measures "d95" distance of L51.start L54.start
  measures "d96" distance of L53.end L60.end
  measures "d97" diameter of A28
  measures "d98" diameter of A27
  measures "d99" diameter of A19
  measures "d100" diameter of A18
  measures "d101" diameter of A26
  measures "d102" distance of L52.start L57.start
  measures "d103" distance of A16.centre L52.start
  measures "d104" distance of A16.centre L45.end
  measures "d105" diameter of A25
  measures "d106" diameter of A16
  measures "d107" diameter of A21
  measures "d108" diameter of A17
  measures "d109" diameter of A15
  measures "d110" diameter of A24
  measures "d111" diameter of A23
  measures "d112" distance of A20.centre L55.end
  measures "d113" distance of L55.end L55.start
  measures "d114" radius of A32
  measures "d115" distance of L71.end L71.start
  measures "d116" distance of A30.centre L80.end
  measures "d117" distance of L71.end L71.start
  measures "d118" distance of L80.end A30.centre
  measures "d119" distance of L81.end L84.end
  measures "d120" distance of L78.end A32.start
  measures "d121" distance of L72.start L74.end
  measures "d122" diameter of A33
  measures "d123" diameter of A42
  measures "d124" diameter of A39
  measures "d125" diameter of A30
  measures "d126" diameter of A43
  measures "d127" distance of L76.start L73.start
  measures "d128" distance of L73.start L73.end
  measures "d129" distance of L73.end A31.centre
  measures "d130" diameter of A35
  measures "d131" diameter of A41
  measures "d132" diameter of A31
  measures "d133" diameter of A36
  measures "d134" diameter of A40
  measures "d135" diameter of A44
  measures "d136" diameter of A34
  measures "d137" distance of A37.centre A32.centre
  measures "d138" distance of L96.start A32.centre
  measures "d194" distance of L102.start L104.end
  measures "d195" distance of L107.start L106.end
  measures "d196" distance of L106.start L106.end
  measures "d203" radius of A50
  measures "d204" diameter of A54
  measures "d205" diameter of A52
  measures "d206" diameter of A55
  measures "d207" diameter of A46
  measures "d208" diameter of A48
  measures "d209" diameter of A47
  measures "d210" diameter of A57
  measures "d211" diameter of A51
  measures "d212" diameter of A45
  measures "d213" diameter of A58
  measures "d214" diameter of A49
  measures "d215" diameter of A53
  measures "d216" distance of L121.end L139.end
  measures "d217" distance of L130.start L135.start
  measures "d218" distance of L121.end L137.end
  measures "d219" distance of L115.start L113.end
  measures "d220" distance of P0 P1
  measures "d350" distance of L157.end L157.start
  measures "d352" distance of L165.start L162.end
  measures "d357" distance of L156.end L167.end
  measures "d358" distance of L156.start L168.end
  measures "d359" distance of L157.end L169.end
  measures "d360" distance of L157.start L170.end
  measures "d361" distance of L176.start L172.start
  measures "d362" distance of L176.start L178.end
  measures "d363" distance of L175.start L179.end
  measures "d364" distance of L171.start L171.end
  measures "d365" distance of L172.start L172.end
  measures "d366" distance of L176.start L184.end
  measures "d367" distance of L178.end L181.end
  measures "d368" radius of A60
  measures "d369" radius of A61
  measures "d370" radius of A62
  measures "d371" radius of A63
  measures "d372" radius of A64
  measures "d373" radius of A65
  measures "d374" radius of A66
  measures "d375" radius of A67
  measures "d376" diameter of A68
  measures "d377" diameter of A69
  measures "d378" diameter of A70
  measures "d379" diameter of A71
  measures "d380" diameter of A72
  measures "d381" diameter of A73
  measures "d382" diameter of A74
  measures "d383" diameter of A75
  measures "d384" distance of L30.end L186.end
  measures "d385" distance of L30.end L188.end
  measures "d387" distance of L31.end L192.end
  measures "d389" distance of L32.end L196.end
  measures "d390" distance of L30.start L198.end
  measures "d391" distance of L30.start L200.end
  measures "d392" diameter of A76
  measures "d393" diameter of A77
  measures "d394" diameter of A78
  measures "d395" diameter of A79
  measures "d537" distance of L30.start L30.end
  measures "d553" distance of L202.start L204.end
  measures "d554" distance of L206.start L208.end
  measures "d555" distance of L210.start L212.end
  measures "d556" distance of L214.start L216.end
  measures "d1" distance of P10 P11
  measures "d2" distance of P9 P10
  measures "d3" radius of A82
  measures "d4" radius of A89
  measures "d5" radius of A85
  measures "d6" radius of A88
  measures "d7" radius of A90
  measures "d8" radius of A80
  measures "d9" radius of A83
  measures "d10" radius of A84
  measures "d597" diameter of A104
  measures "d598" diameter of A111
  measures "d599" diameter of A110
  measures "d600" diameter of A113
  measures "d601" diameter of A106